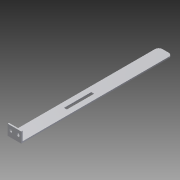
# Autodesk Inventor part: Fork 3 ver2c
Saved by Autodesk Inventor 2015 (Build 190159000, 159)
## iProperties
Created: 2015-06-22
Part Number: Fork 3 ver2c
Material: アルミニウム 5052 H32
Document SubType Name: Modeling
Designer: kenta
Density: 2.68 g/cm^3
Appearance: サテン
Mass: 10.1507 g
Surface Area: 57.4644 cm^2
Volume: 3.78756 cm^3
Author: kenta
Autodesk Inventor part; units mm, degrees
ref_plane "YZ Plane" through (0, 0, 0) normal (1, 0, 0) x (0, 1, 0)
ref_plane "XZ Plane" through (0, 0, 0) normal (0, 1, 0) x (-1, 0, 0)
ref_plane "XY Plane" through (0, 0, 0) normal (0, 0, 1) x (1, 0, 0)
sketch "スケッチ1" plane through (0, 0, 0) normal (0, 0, 1) x (1, 0, 0)
  line L0 (-7.5, 83) -> (7.5, 83)
  line L1 (7.5, 83) -> (7.5, -83)
  line L2 (7.5, -83) -> (-7.5, -83)
  line L3 (-7.5, -83) -> (-7.5, 83)
  line L4 (-7.5, 83) -> (7.5, -83) construction
  line L5 (7.5, 83) -> (-7.5, -83) construction
  point P0 (0, 0)
  dimension "d0" = 15
  dimension "d1" = 166
  constraints: 12 end point, 2 midpoint, 2 parallel, 1 horizontal, 1 perpendicular
  measures "d0" distance of L1.end L2.end
  measures "d1" distance of L2.end L0.start
extrude "押し出し1" add sketch "スケッチ1" along normal blind 1.5
sketch "スケッチ2" plane through (0, 0, 1.5) normal (0, 0, 1) x (1, 0, 0)
  line L0 (7.5, 83) -> (-7.5, 83) projected
  line L1 (-1.55, 3) -> (1.55, 3)
  line L2 (1.55, 3) -> (1.55, -27)
  line L3 (1.55, -27) -> (-1.55, -27)
  line L4 (-1.55, -27) -> (-1.55, 3)
  line L5 (-7.5, 83) -> (-7.5, -83) projected
  point P0 (0, 0)
  dimension "d6" = 3.1
  dimension "d7" = 30
  dimension "d8" = 80
  dimension "d9" = 5.95
  constraints: 8 end point, 2 parallel, 1 horizontal, 1 perpendicular
  measures "d6" distance of L2.end L3.end
  measures "d7" distance of L1.end L2.end
  measures "d8" distance between parallel lines of L1 L0
  measures "d9" distance between parallel lines of L4 L5
extrude "押し出し2" cut sketch "スケッチ2" against normal blind 1.5
sketch "スケッチ3" plane through (0, 0, 1.5) normal (0, 0, 1) x (1, 0, 0)
  line L0 (-7.5, -83) -> (7.5, -83)
  line L1 (7.5, -83) -> (7.5, -81.5)
  line L2 (7.5, -81.5) -> (-7.5, -81.5)
  line L3 (-7.5, -81.5) -> (-7.5, -83)
  point P0 (0, 0)
  dimension "d12" = 1.5
  constraints: 8 end point, 2 parallel, 1 horizontal, 1 perpendicular
  measures "d12" distance of L1.end L0.end
extrude "押し出し3" add sketch "スケッチ3" along normal blind 10
sketch "スケッチ4" plane through (-7.5, -81.5, 1.5) normal (0, 1, 0) x (1, 0, 0)
  line L0 (15, -10) -> (0, -10) projected
  line L1 (15, 0) -> (15, -10) projected
  point P0 (7.5, 1.5)
  point P1 (11.5, -5)
  point P2 (3.5, -5)
  dimension "d15" = 8
  dimension "d16" = 5
  dimension "d17" = 3.5
  constraints: 1 horizontal alignment
  measures "d15" distance of point (3.5, -5) point (11.5, -5)
  measures "d16" distance from line of point (11.5, -5) L0
  measures "d17" distance from line of L1 point (11.5, -5)
hole "穴1" at (4, -81.5, 6.5) at (-4, -81.5, 6.5) direction (0, -1, 0) diameter 3.1 end through all
fillet "フィレット1" radius 4 2 edges at (-7.5, 83, 0.75) (7.5, 83, 0.75)
